Autodesk Inventor part; units mm, degrees
(part 2 of 2)
extrude "Extrusion1" add sketch "Sketch1" along normal blind 0.25 contours L127 L128 L129 L130 L131 L132 L133 L134 L135 L136 L137 L138 L139 L140 L141 L142 L143 L144 L145 L146 L147 L148 L149 L150 L151 L152 L153 L154 L155 L156 L157 L158 L159 L160 L161 L162 L163 L164 L165 L166 L167 L168 L169 L170 L171 L172 L173 L174 L175 L176 L177 L178 L179 L180 L181 L182 L183 L184 L185 L186 L187 L188 L189 L190 L191 L192 L193 L194 L195 L196 L197 L198 | L720 L719 L718 L717 L716 L715 L714 L713 L712 L711 L710 L709 L708 L707 L706 L705 L704 L703 L702 L701 L700 L699 L698 L697 L696 L695 L694 L693 L692 L691 L690 L689 L688 L687 L686 L685 L683 L682 L681 L680 L679 L678 L677 L676 L675 L674 L673 L672 L671 L670 L669 L668 L667 L666 L665 L664 L663 L662 L661 L660 L659 L658 L657 L656 L655 L654 L653 L652 L651 L650 L649 L648
extrude "Extrusion2" add sketch "Sketch1" along normal blind 0.5 contours L199 L200 L201 L202 L203 L204 L205 L206 L207 L208 L209 L210 L211 L212 L213 L214 L215 L216 L217 L218 L219 L220 L221 L222 L223 L224 L225 L226 L227 L228 L229 L230 L231 L232 L233 L234 L235 L236 L237 L238 | L890 L883 L885 L240 | L240 L885 L884 L890 | L885 L883 L243 L240 | L240 L243 L884 L885 | L243 L883 L886 L240 | L240 L886 L884 L243 | L884 L243 L888 L885 | L885 L889 L243 L883 | L886 L883 L887 L240 | L240 L887 L884 L886 | L884 L886 L888 L243 | L243 L889 L886 L883 | L245 L246 L247 L248 L249 L250 L251 L252 L253 L254 L255 L256 L257 L258 L259 L260 L261 L262 L263 L264 L265 L266 L267 L268 L269 L270 L271 L272 L273 L274 L275 L276 L277 L278 L279 L280 L281 L282 L283 L284 L285 L286 L287 L288 L289 L290 L291 L292 L293 L294 L295 L296 L297 L298 L299 L300 L301 L302 L303 L304 L305 L306 L307 L308 L309 L310 L311 L312 L313 L314 L315 L316 L317 L318 L319 L320 L321 L322 L323 L324 L325 L326 L327 L328 L329 L330 L331 L332 L333 L334 L335 L336 L337 L338 L339 L340 L341 L342 L343 L344 L345 L346 L347 L348 L349 L350 L351 L352 L353 L354 L355 L356 L357 L358 L359 L360 L361 L362 L363 L364 L365 L366 L367 L368 L369 L370 L371 L372 L373 L374 L375 L376 L377 L378 L379 L380 L381 L382 L383 L384 L385 L386 L387 L388 L389 L390 L391 L392 L393 L394 L395 L396 L397 L398 L399 L400 L401 L402 L403 L404 L405 L406 L407 L408 L409 L410 L411 L412 L413 L414 L415 L416 L417 L418 L419 L420 L421 L422 L423 L424 L425 L426 L427 L428 L429 L430 L431 L432 L433 L434 L435 L436 L437 L438 L439 L440 L441 L442 L443 L444 L445 L446 L447 L448 L449 L450 L451 L452 L453 L454 L455 L456 L457 L458 L459 L460 L461 L462 L463 L464 L465 L466 L467 L468 L469 L470 L471 L472 L473 L474 L475 L476 L477 L478 L479 L480 L481 L482 L483 L484 L485 L486 L487 L488 L489 L490 L491 L492 L493 L494 L495 L496 L497 L498 L499 L500 L501 L502 L503 L504 L505 L506 L507 L508 L509 L510 L511 L512 L513 L514 L515 L516 L517 L518 L519 L520 L521 L522 L523 L524 L525 L526 L527 L528 L529 L530 L531 L532 L533 L534 L535 L536 L537 L538 L539 L540 L541 L542 L543 L544 L545 L546 L547 L548 L549 L550 L551 L552 L553 L554 L555 L556 L557 L558 L559 L560 L561 L562 L563 L564 L565 L566 L567 L568 L569 L570 L571 L572 L573 L574 L575 L576 L577 L578 L579 L580 L581 L582 L583 L584 L585 L586 L587 L588 L589 L590 L591 L592 L593 L594 L595 L596 L597 L598 L599 L600 L601 L602 L603 L604 L605 L606 L607 L608 L609 L610 L611 L612 L613 L614 L615 L616 L617 L618 L619 L620 L621 L622 L623 L624 L625 L626 L627 L628 L629 L630 L631 L632 L633 L634 L635 L636 L637 L638 L639 L640 L641 L642 L643 L644 L645 L646
extrude "Extrusion3" cut sketch "Sketch1" along normal through all both and the other way through all contours L890 L883 L885 L240 | L240 L885 L884 L890 | L885 L883 L243 L240 | L240 L243 L884 L885 | L243 L883 L886 L240 | L240 L886 L884 L243 | L884 L243 L888 L885 | L885 L889 L243 L883 | L886 L883 L887 L240 | L240 L887 L884 L886 | L884 L886 L888 L243 | L243 L889 L886 L883
body "Solid1"
